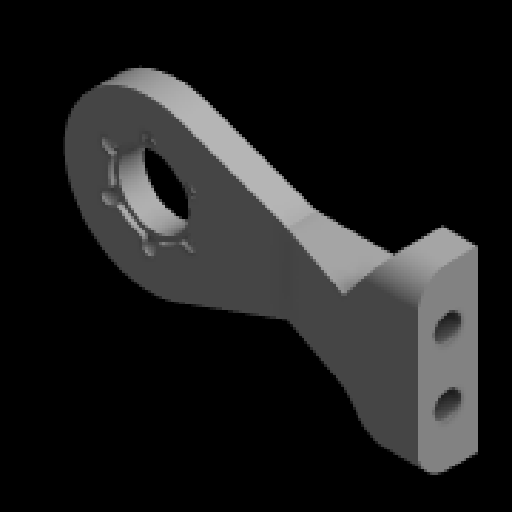
# Autodesk Inventor part: NeckMount
Saved by Autodesk Inventor 2025.2 (Build 292293000, 293)
## iProperties
Created: 2026-01-12
Part Number: NeckMount
Material: Generic
Document SubType Name: Modeling
Designer: valer
Density: 1 g/cm^3
Appearance: Default
Author: valer
Autodesk Inventor part; units mm, degrees
ref_plane "YZ Plane" through (0, 0, 0) normal (1, 0, 0) x (0, 1, 0)
ref_plane "XZ Plane" through (0, 0, 0) normal (0, 1, 0) x (-1, 0, 0)
ref_plane "XY Plane" through (0, 0, 0) normal (0, 0, 1) x (1, 0, 0)
sketch "Base" plane through (0, 0, 0) normal (0, 0, 1) x (1, 0, 0)
  circle A0 centre (0, 0) radius 7
  circle A1 centre (0, 0) radius 17
  line L0 (-32.4, 0) -> (75.4, 0) construction
  line L1 (5.8143, 15.9748) -> (27.7249, 8)
  line L2 (27.7249, 8) -> (45.1871, 8)
  line L3 (45.1871, 8) -> (53, 18)
  line L4 (53, 18) -> (60, 18)
  line L5 (60, 18) -> (60, 0)
  line L6 (5.8143, -15.9748) -> (27.7249, -8)
  line L7 (27.7249, -8) -> (45.1871, -8)
  line L8 (45.1871, -8) -> (53, -18)
  line L9 (53, -18) -> (60, -18)
  line L10 (60, -18) -> (60, 0)
  point P0 (5.8143, -15.9748)
  dimension "d1" = 34
  dimension "d0" = 14
  dimension "d2" = 18
  dimension "d3" = 128
  dimension "d4" = 7
  dimension "d6" = 160
  dimension "d7" = 60
  dimension "d8" = 16
  constraints: 20 end point, 5 symmetric about line, 2 coincident, 1 centre point, 1 horizontal, 1 parallel, 1 perpendicular, 1 point on line, 4 other
  measures "d0" diameter of A0
  measures "d2" distance of L4.end L5.end
  measures "d3" angle of L4 L3
  measures "d4" distance of L3.end L4.end
  measures "d6" angle of L2 L1
  measures "d7" distance from line of L5 point (0, 0)
  measures "d8" distance between parallel lines of L7 L2
extrude "BaseFeature" add sketch "Base" along normal mid plane 6
sketch "Mount" plane through (0, 0, 3) normal (0, 0, 1) x (1, 0, 0)
  line L0 (60, 18) -> (53, 18) projected
  line L1 (60, -18) -> (60, 18) projected
  line L2 (53, -18) -> (60, -18) projected
  line L3 (45.1871, -8) -> (53, -18) projected
  line L4 (53, 18) -> (45.1871, 8) projected
  line L5 (45.1871, 8) -> (45.1871, -8)
  point P0 (0, 0)
  constraints: 2 end point, 1 vertical
extrude "MountFeature" add sketch "Mount" along normal blind 6
sketch "MountTransition" plane through (27.7249, -8, -3) normal (0, -1, 0) x (1, 0, 0)
  line L0 (0, 6) -> (17.4623, 6) projected
  line L1 (0, 6) -> (17.4623, 12)
  line L2 (17.4623, 6) -> (17.4623, 12) projected
  point P0 (-27.7249, 3)
  constraints: 2 end point
extrude "MountTransitionFeature" add sketch "MountTransition" against normal up to surface (16 mm away)
fillet "MountFilletsFeature" radius 6 2 edges at (56.5, 18, 9) (56.5, -18, 9)
sketch "MountHoles" plane through (60, -12, 9) normal (1, 0, 0) x (0, 0, -1)
  arc A0 (6, 30) -> (0, 24) centre (6, 24) ccw construction
  line L0 (12, 30) -> (12, -6) projected
  arc A1 (0, 0) -> (6, -6) centre (6, 0) ccw construction
  line L1 (6, 24) -> (6, 0) construction
  circle A2 centre (6, 18.7) radius 3
  line L2 (12, 12) -> (0, 12) construction
  line L3 (0, 0) -> (0, 24) projected
  circle A3 centre (6, 5.3) radius 3
  dimension "d56" = 6
  dimension "d57" = 13.4
  constraints: 4 end point, 2 centre point, 2 midpoint, 1 point on line, 1 symmetric about line, 1 vertical, 1 other
  measures "d56" diameter of A2
  measures "d57" distance of A3.centre A2.centre
sketch "HubMount" plane through (0, 0, 3) normal (0, 0, 1) x (1, 0, 0)
  circle A0 centre (0, -9.525) radius 1.25 projected
  circle A1 centre (8.2489, -4.7625) radius 1.25 projected
  circle A2 centre (8.2489, 4.7625) radius 1.25 projected
  circle A3 centre (0, 9.525) radius 1.25 projected
  circle A4 centre (-8.2489, 4.7625) radius 1.25 projected
  circle A5 centre (-8.2489, -4.7625) radius 1.25 projected
  point P0 (0, 0)
extrude "HubMountFeature" cut sketch "HubMount" against normal through all
sketch "BearingIndentation" plane through (0, 0, 3) normal (0, 0, 1) x (1, 0, 0)
  circle A0 centre (0, 0) radius 7 projected
  circle A1 centre (0, 0) radius 8.05
  circle A2 centre (0, 9.525) radius 1.25 projected
  circle A3 centre (8.2489, 4.7625) radius 1.25 projected
  circle A4 centre (-8.2489, 4.7625) radius 1.25 projected
  circle A5 centre (-8.2489, -4.7625) radius 1.25 projected
  circle A6 centre (0, -9.525) radius 1.25 projected
  circle A7 centre (8.2489, -4.7625) radius 1.25 projected
  line L0 (-8.2489, 4.7625) -> (0, 0) construction
  line L1 (0, 9.525) -> (0, 0) construction
  line L2 (-7.6239, 5.845) -> (-6.2619, 5.0587)
  line L3 (-8.8739, 3.68) -> (-7.5119, 2.8936)
  line L4 (-1.25, 9.525) -> (-1.25, 7.9524)
  line L5 (1.25, 9.525) -> (1.25, 7.9524)
  line L6 (7.6239, 5.845) -> (6.2619, 5.0587)
  line L7 (8.8739, 3.68) -> (7.5119, 2.8936)
  line L8 (-32.4, 0) -> (75.4, 0) construction
  line L9 (-7.6239, -5.845) -> (-6.2619, -5.0587)
  line L10 (-8.8739, -3.68) -> (-7.5119, -2.8936)
  line L11 (-1.25, -9.525) -> (-1.25, -7.9524)
  line L12 (1.25, -9.525) -> (1.25, -7.9524)
  line L13 (7.6239, -5.845) -> (6.2619, -5.0587)
  line L14 (8.8739, -3.68) -> (7.5119, -2.8936)
  point P0 (1.25, -9.525)
  dimension "d47" = 16.1
  constraints: 28 end point, 16 symmetric about line, 8 point on circle, 4 tangent, 3 parallel, 2 vertical, 1 centre point, 1 coincident
  measures "d47" diameter of A1
extrude "BearingIndentationFeature" cut sketch "BearingIndentation" against normal blind 1 contours A1 | A1 L6 A3 L7 | L14 A7 L13 A1 | A1 L4 A2 L5 | L12 A6 L11 A1 | A1 L3 A4 L2 | L9 A5 L10 A1
fillet "BearingIndentationFilletsFeature" radius 1 11 edges at (-6.2619, 5.0587, 2.5) (-1.25, 7.9524, 2.5) (1.25, 7.9524, 2.5) (6.2619, 5.0587, 2.5) (-7.5119, -2.8936, 2.5) (-6.2619, -5.0587, 2.5) (-1.25, -7.9524, 2.5) (1.25, -7.9524, 2.5) (6.2619, -5.0587, 2.5) (7.5119, -2.8936, 2.5) (7.5119, 2.8936, 2.5)
hole "MountHolesFeature" at (60, 6.7, 3) at (60, -6.7, 3) direction (-1, 0, 0) diameter 5.4 depth 11 tip angle 118
body "Solid1"
